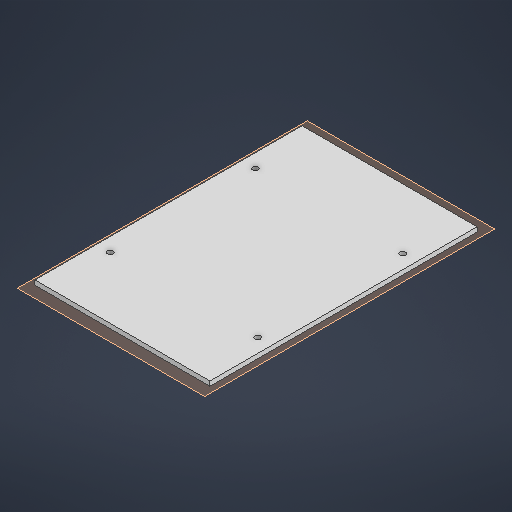
# Autodesk Inventor part: bed_plate
Saved by Autodesk Inventor 2025 (Build 290162000, 162)
## iProperties
Created: 2024-06-24
Part Number: bed_plate
Material: Generic
Document SubType Name: Modeling
Designer: Windows 7 was better
Density: 1 g/cm^3
Appearance: Default
Author: Windows 7 was better
Autodesk Inventor part; units mm, degrees
ref_plane "YZ Plane" through (0, 0, 0) normal (1, 0, 0) x (0, 1, 0)
ref_plane "XZ Plane" through (0, 0, 0) normal (0, 1, 0) x (-1, 0, 0)
ref_plane "XY Plane" through (0, 0, 0) normal (0, 0, 1) x (1, 0, 0)
ref_plane "Work Plane1" through (-51.3814, -5.3745, -158.8704) normal (0, 1, 0) x (1, 0, 0)
sketch "Sketch1" plane through (-51.3814, -5.3745, -158.8704) normal (0, 1, 0) x (1, 0, 0)
  line L0 (74, 114.5) -> (74, 71.5) projected
  line L1 (-74, 114.5) -> (74, 114.5) projected
  line L2 (-74, 71.5) -> (-74, 114.5) projected
  line L3 (-64, 71.5) -> (-74, 71.5) projected
  arc A0 (-64, 55.5) -> (-64, 71.5) centre (-64, 63.5) ccw projected
  line L4 (-74, 55.5) -> (-64, 55.5) projected
  line L5 (-74, -54.5) -> (-74, 55.5) projected
  line L6 (-64, -54.5) -> (-74, -54.5) projected
  arc A1 (-64, -70.5) -> (-64, -54.5) centre (-64, -62.5) ccw projected
  line L7 (-74, -70.5) -> (-64, -70.5) projected
  line L8 (-74, -114.5) -> (-74, -70.5) projected
  line L9 (74, -114.5) -> (-74, -114.5) projected
  line L10 (74, -70.5) -> (74, -114.5) projected
  line L11 (64, -70.5) -> (74, -70.5) projected
  arc A2 (64, -54.5) -> (64, -70.5) centre (64, -62.5) ccw projected
  line L12 (74, -54.5) -> (64, -54.5) projected
  line L13 (74, 55.5) -> (74, -54.5) projected
  line L14 (64, 55.5) -> (74, 55.5) projected
  arc A3 (64, 71.5) -> (64, 55.5) centre (64, 63.5) ccw projected
  line L15 (74, 71.5) -> (64, 71.5) projected
  line L16 (0, 114.5) -> (0, -114.5) construction
  line L17 (-76, 116) -> (76, 116)
  line L18 (76, 116) -> (76, -116)
  line L19 (76, -116) -> (-76, -116)
  line L20 (-76, -116) -> (-76, 116)
  line L21 (-76, 116) -> (76, -116) construction
  line L22 (76, 116) -> (-76, -116) construction
  circle A4 centre (-64, -62.5) radius 2.413
  circle A5 centre (-64, 63.5) radius 2.413
  circle A6 centre (64, 63.5) radius 2.413
  circle A7 centre (64, -62.5) radius 2.413
  point P0 (51.3814, -158.8704)
  point P1 (0, 0)
  dimension "d0" = 152
  dimension "d1" = 232
  dimension "d2" = 4.826
  dimension "d3" = 4.826
  dimension "d4" = 4.826
  dimension "d5" = 4.826
  constraints: 14 end point, 5 midpoint, 4 centre point, 4 coincident, 2 parallel, 1 horizontal, 1 perpendicular
  measures "d0" distance of L18.end L19.end
  measures "d1" distance of L17.end L18.end
  measures "d2" diameter of A4
  measures "d3" diameter of A5
  measures "d4" diameter of A6
  measures "d5" diameter of A7
extrude "Extrusion1" add sketch "Sketch1" along normal blind 4 contours L0 L15 A3 L14 L13 L12 A2 L11 L10 L9 L8 L7 A1 L6 L5 L4 A0 L3 L2 L1 | L17 L18 L19 L20
body "Solid1"
